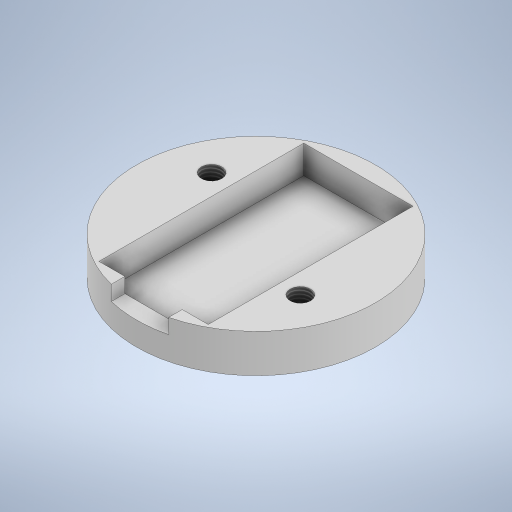
# Autodesk Inventor part: DHT11-Case-Btm
Saved by Autodesk Inventor 2023 (Build 270158000, 158)
## iProperties
Created: 2024-03-03
Part Number: DHT11-Case-Btm
Material: Generic
Document SubType Name: Modeling
Designer: ongyu
Density: 1 g/cm^3
Appearance: Default
Author: ongyu
Autodesk Inventor part; units mm, degrees
ref_plane "YZ Plane" through (0, 0, 0) normal (1, 0, 0) x (0, 1, 0)
sketch "Sketch1" plane through (0, 0, 0) normal (0, 1, 0) x (-1, 0, 0)
  line L0 (8, -15) -> (-8, -15)
  line L1 (-8, -15) -> (-8, 15)
  line L2 (-8, 15) -> (8, 15)
  line L3 (8, 15) -> (8, -15)
  line L4 (-24.5, 0) -> (24.5, 0) projected
  line L5 (0, -24.5) -> (0, 24.5) projected
  circle A0 centre (0, 0) radius 17.5
  line L6 (4.2, 15) -> (4.2, 16.9885)
  line L7 (-4.2, 15) -> (-4.2, 16.9885)
  dimension "d0" = 30
  dimension "d1" = 15
  dimension "d2" = 16
  dimension "d3" = 8
  dimension "d11" = 8.4
  dimension "d12" = 4.2
  dimension "d13" = 35
  constraints: 12 end point, 2 parallel, 2 point on circle, 2 point on line, 2 vertical, 1 centre point, 1 coincident, 1 horizontal, 1 perpendicular
  measures "d0" distance between parallel lines of L2 L0
  measures "d1" distance between parallel lines of L4 L0
  measures "d2" distance between parallel lines of L3 L1
  measures "d3" distance between parallel lines of L3 L5
  measures "d11" distance between parallel lines of L6 L7
  measures "d12" distance between parallel lines of L5 L6
  measures "d13" diameter of A0
extrude "Extrusion1" add sketch "Sketch1" against normal blind 1.5
extrude "Extrusion2" add sketch "Sketch1" along normal blind 8.25 contours L3 L4 A0 L5 L0 | L5 A0 L4 L1 L0 | L3 L2 L6 A0 L4 | L4 A0 L7 L2 L1
extrude "Extrusion4" add sketch "Sketch1" along normal blind 1.94 contours L5 A0 L6 L2 | L2 L7 A0 L5
sketch "Sketch2" plane through (0, 8.25, 0) normal (0, 1, 0) x (1, 0, 0)
  arc A0 (4.2, -16.9885) -> (-4.2, -16.9885) centre (0, 0) ccw projected
  arc A1 (-4.2, -16.9885) -> (4.2, -16.9885) centre (0, 0) ccw projected
extrude "Extrusion5" add sketch "Sketch2" along normal blind 1.5
sketch "Sketch3" plane through (0, 8.25, 0) normal (0, -1, 0) x (1, 0, 0)
  line L0 (4.2, 15) -> (-4.2, 15) projected
  line L1 (4.2, 15) -> (4.2, 16.9885) projected
  arc A0 (4.2, 16.9885) -> (-4.2, 16.9885) centre (0, 0) ccw projected
  line L2 (-4.2, 16.9885) -> (-4.2, 15) projected
extrude "Extrusion6" add sketch "Sketch3" along normal blind 1.25
sketch "Sketch4" plane through (0, 7, 0) normal (0, -1, 0) x (1, 0, 0)
  line L0 (-3.9, 17.9983) -> (-3.9, 11.1923)
  line L1 (-4.2, 16.9885) -> (-4.2, 15) projected
  line L2 (3.9, 18.3816) -> (3.9, 12.4257)
  line L3 (4.2, 15) -> (4.2, 16.9885) projected
  line L4 (2.7, 18.3816) -> (2.7, 12.4257)
  line L5 (-2.7, 17.9983) -> (-2.7, 11.1923)
  arc A0 (4.2, 16.9885) -> (-4.2, 16.9885) centre (0, 0) ccw projected
  line L6 (-4.2, 15) -> (4.2, 15) projected
  point P0 (2.7, 15)
  point P1 (3.9, 15)
  point P2 (3.9, 17.0599)
  point P3 (2.7, 17.2905)
  point P4 (-3.9, 15)
  point P5 (-2.7, 15)
  point P6 (-2.7, 17.2905)
  point P7 (-3.9, 17.0599)
  dimension "d22" = 0.3
  dimension "d23" = 0.3
  dimension "d24" = 1.2
  dimension "d25" = 1.2
  constraints: 8 end point, 2 parallel, 2 vertical
  measures "d22" distance between parallel lines of L1 L0
  measures "d23" distance between parallel lines of L3 L2
  measures "d24" distance between parallel lines of L2 L4
  measures "d25" distance between parallel lines of L0 L5
extrude "Extrusion7" cut sketch "Sketch4" against normal blind 1.2 contours A0 L5 L6 L0 | A0 L2 L6 L4
ref_plane "Work Plane1" through (0, 9.75, 0) normal (0, 1, 0) x (1, 0, 0)
sketch "Sketch5" plane through (0, 9.75, 0) normal (0, 1, 0) x (1, 0, 0)
  line L0 (-6, 25.5522) -> (6, 25.5522)
  line L1 (-5.75, 13.625) -> (-5.75, -1.375)
  line L2 (5.75, 13.625) -> (5.75, -1.375)
  line L3 (-5.75, -1.375) -> (5.75, -1.375)
  line L4 (-5.75, 13.625) -> (5.75, 13.625)
  line L5 (-4.75, 12.625) -> (4.75, 12.625)
  line L6 (4.75, 12.625) -> (4.75, -0.375)
  line L7 (4.75, -0.375) -> (-4.75, -0.375)
  line L8 (-4.75, -0.375) -> (-4.75, 12.625)
  line L9 (0, 30.9376) -> (0, -6.7604) projected
  point P0 (0, 0)
  dimension "d29" = 12
  dimension "d32" = 15
  dimension "d37" = 0
  dimension "d38" = 0
  dimension "d39" = 1
  dimension "d40" = 1
  dimension "d44" = 5.75
  dimension "d45" = 11.5
  dimension "d46" = 0
  dimension "d47" = 0
  constraints: 18 end point, 2 horizontal, 2 point on line, 2 vertical, 1 parallel, 1 perpendicular, 2 other
  measures "d29" distance of L0.start L0.end
  measures "d32" distance of L1.start L1.end
  measures "d37" distance from line of L4 L2.start
  measures "d38" distance from line of L4 L1.start
  measures "d39" distance between parallel lines of L4 L5
  measures "d40" distance between parallel lines of L2 L6
  measures "d44" distance between parallel lines of L9 L2
  measures "d45" distance between parallel lines of L1 L2
  measures "d46" distance of L6.start L5.end
  measures "d47" distance from line of L8 L5.start
extrude "Extrusion9" cut sketch "Sketch5" against normal up to surface (1.5 mm away) contours L9 L7 L8 L5 | L5 L6 L7 L9
ref_plane "Work Plane2" through (0, 7, 0) normal (0, -1, 0) x (1, 0, 0)
fillet "Fillet3" radius 1.5 1 edges at (4.2, 9.75, -16.9885)
fillet "Fillet4" radius 1.5 4 edges at (0, 9.75, -12.625) (4.75, 9.75, -6.125) (-4.75, 9.75, -6.125) (0, 9.75, 0.375)
sketch "Sketch6" plane through (0, 0, 0) normal (0, 0, 1) x (1, 0, 0)
  line L0 (-25.8332, 4.125) -> (28.0495, 4.125)
  line L1 (-16, 9.75) -> (16, 9.75) projected
  line L2 (-8, 0) -> (8, 0) projected
  line L3 (19.5176, 4.125) -> (-21.0233, 4.125)
  line L4 (-21.0233, 4.125) -> (-21.0233, 9.75)
  line L5 (-21.0233, 9.75) -> (19.5176, 9.75)
  line L6 (19.5176, 9.75) -> (19.5176, 4.125)
  line L7 (-17.5, -1.5) -> (17.5, -1.5) projected
  point P0 (0, 0)
  point P1 (16, 9.75)
  point P2 (-16, 9.75)
  point P3 (-21.0233, 4.125)
  dimension "d53" = 5.625
  dimension "d72" = 11.25
  constraints: 10 end point, 2 horizontal, 2 parallel, 1 perpendicular, 1 point on line
  measures "d53" distance between parallel lines of L0 L1
  measures "d72" distance between parallel lines of L7 L1
extrude "Extrusion10" cut sketch "Sketch6" against normal blind 30.25
extrude "Extrusion11" cut sketch "Sketch6" along normal blind 27.125
sketch "Sketch7" plane through (0, 4.125, 0) normal (0, 1, 0) x (1, 0, 0)
  circle A0 centre (-11, 4.5) radius 1.5
  circle A1 centre (11, -4.5) radius 1.5
  line L0 (8, -15) -> (8, 15) projected
  line L1 (-8, 15) -> (-8, -15) projected
  line L2 (0, 24.5) -> (0, -24.5) projected
  point P0 (0, 0)
  dimension "d60" = 3
  dimension "d61" = 3
  dimension "d62" = 3
  dimension "d63" = 3
  dimension "d64" = 4.5
  dimension "d65" = 4.5
  dimension "d73" = 11
  dimension "d74" = 11
  constraints: 2 centre point
  measures "d60" diameter of A0
  measures "d61" diameter of A1
  measures "d62" distance from line of L0 A1.centre
  measures "d63" distance from line of L1 A0.centre
  measures "d64" vertical distance of point (0, 0) A0.centre
  measures "d65" vertical distance of point (0, 0) A1.centre
  measures "d73" distance from line of L2 A0.centre
  measures "d74" distance from line of L2 A1.centre
extrude "Extrusion12" cut sketch "Sketch7" against normal blind 2.5
thread "Thread1" size "M3x0.5" class "6H" standard "ANSI Metric M Profile" length 9
thread "Thread2" size "M3x0.5" class "6H" standard "ANSI Metric M Profile" length 9
sketch "Sketch8" plane through (0, -1.5, 0) normal (0, -1, 0) x (1, 0, 0)
  line L0 (15, -1) -> (-15, -1)
  line L1 (-15, -1) -> (-15, 1)
  line L2 (-15, 1) -> (15, 1)
  line L3 (15, 1) -> (15, -1)
  line L4 (-24.5, 0) -> (24.5, 0) projected
  line L5 (0, 24.5) -> (0, -24.5) projected
  line L6 (2.5, 5) -> (-2.5, 5)
  line L7 (-2.5, 5) -> (-2.5, -5)
  line L8 (-2.5, -5) -> (2.5, -5)
  line L9 (2.5, -5) -> (2.5, 5)
  point P0 (0, 0)
  point P1 (2.5, -1)
  point P2 (-2.5, -1)
  point P3 (2.5, 1)
  point P4 (-2.5, 1)
  dimension "d75" = 30
  dimension "d76" = 2
  dimension "d77" = 1
  dimension "d78" = 15
  dimension "d81" = 10
  dimension "d82" = 5
  dimension "d83" = 5
  dimension "d84" = 2.5
  constraints: 16 end point, 4 parallel, 2 horizontal, 2 perpendicular
  measures "d75" distance between parallel lines of L1 L3
  measures "d76" distance between parallel lines of L2 L0
  measures "d77" distance between parallel lines of L4 L0
  measures "d78" distance between parallel lines of L3 L5
  measures "d81" distance between parallel lines of L6 L8
  measures "d82" distance between parallel lines of L6 L4
  measures "d83" distance between parallel lines of L7 L9
  measures "d84" distance between parallel lines of L5 L9
extrude "Extrusion13" cut sketch "Sketch8" against normal blind 1 contours L0 L9 L4 L3 | L0 L5 L4 L9 | L4 L9 L2 L3 | L0 L7 L4 L5 | L4 L5 L2 L9 | L0 L1 L4 L7 | L4 L7 L2 L5 | L4 L1 L2 L7
extrude "Extrusion14" cut sketch "Sketch8" against normal blind 0.5 contours L9 L8 L5 L0 | L5 L8 L7 L0 | L2 L5 L6 L9 | L2 L7 L6 L5
equation "\"d1\" = 0.5 * d0"
equation "\"d3\" = 0.5 * d2"
equation "\"d12\" = 0.5 * d11"
equation "\"d23\" = d22"
equation "\"d25\" = d24"
equation "\"d44\" = 0.5 * d45"
equation "\"d53\" = 0.5 * d72"
equation "\"d65\" = d64"
equation "\"d77\" = 0.5 * d76"
equation "\"d78\" = 0.5 * d75"
equation "\"d82\" = 0.5 * d81"
equation "\"d84\" = 0.5 * d83"
body "Solid1"
